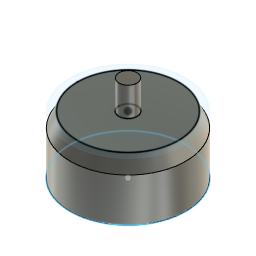
motor v2 (Autodesk Fusion 360 design; units mm, degrees)
Autodesk Fusion 360 part; units mm, degrees
sketch "Sketch1" plane through (0, 0, 0) normal (0, 0, 1) x (1, 0, 0)
  circle A0 centre (0.4513, 0) radius 4
  dimension "d1" = 8
  measures "d1" diameter of A0
extrude "Extrude1" add sketch "Sketch1" along normal blind 4
sketch "Sketch2" plane through (0, 0, 4) normal (0, 0, 1) x (-1, 0, 0)
  circle A0 centre (-0.4513, 0) radius 4
  circle A1 centre (-0.4513, 0) radius 3.5
  circle A2 centre (-0.4513, 0) radius 0.625
  dimension "d4" = 7
  dimension "d5" = 1.25
  constraint concentric A0 A1
  constraint concentric A1 A2
  measures "d4" diameter of A1
  measures "d5" diameter of A2
extrude "Extrude2" cut 1 faces at (2.3843, -0.8657, 4) along direction (0, 0, -1) blind 1
loft "Loft1" add profiles "Sketch2" section 1 face at (2.3843, -0.8657, 3) section 2 contours A1
extrude "Extrude3" add sketch "Sketch2" along normal blind 2 contours A2
